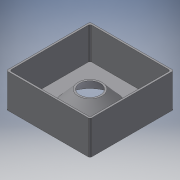
# Autodesk Inventor part: contenção
Saved by Autodesk Inventor 2019.4 (Build 234330000, 330)
## iProperties
Created: 2019-10-16
Part Number: contenção
Material: Genérico
Document SubType Name: Modeling
Designer: natha
Density: 1 g/cm^3
Appearance: Padrão
Author: natha
Autodesk Inventor part; units mm, degrees
ref_plane "YZ Plane" through (0, 0, 0) normal (1, 0, 0) x (0, 1, 0)
ref_plane "XY Plane" through (0, 0, 0) normal (0, 0, 1) x (1, 0, 0)
sketch "Esboço1" plane through (0, 0, 0) normal (0, 1, 0) x (-1, 0, 0)
  line L0 (-49, 49) -> (49, 49)
  line L1 (49, 49) -> (49, -49)
  line L2 (49, -49) -> (-49, -49)
  line L3 (-49, -49) -> (-49, 49)
  line L4 (-49, 49) -> (49, -49) construction
  line L5 (49, 49) -> (-49, -49) construction
  point P0 (0, 0)
  dimension "d0" = 98
  dimension "d1" = 98
  constraints: 12 end point, 2 midpoint, 2 parallel, 1 horizontal, 1 perpendicular
  measures "d0" distance of L0.end L1.end
  measures "d1" distance of L1.end L2.end
extrude "Extrusão1" add sketch "Esboço1" along normal blind 39.4
shell "Casca1" thickness 2 removed faces 1 at (16.3333, 39.4, 16.3333)
sketch "Esboço3" plane through (0, 0, 0) normal (0, 0, 1) x (1, 0, 0)
  line L0 (0, 0) -> (32, 0)
  line L1 (49, 0) -> (-49, 0) projected
  line L2 (32, 0) -> (0, 36.5533)
  line L3 (0, 0) -> (0, 36.5533)
  point P0 (-43.1, 0)
  dimension "d6" = 32
  dimension "d7" = 48.8
  constraints: 6 end point, 1 point on line, 1 vertical
  measures "d6" distance of L0.start L0.end
  measures "d7" angle of L0 L2
revolve "Revolução1" add sketch "Esboço3" angle 360 about axis through (0, 0, 0) along (0, 1, 0)
sketch "Esboço4" plane through (0, 0, 0) normal (0, 0, 1) x (1, 0, 0)
  line L0 (0, 0) -> (30, 0)
  line L1 (-49, 0) -> (49, 0) projected
  line L2 (0, 36.5533) -> (-30.2491, 2) projected
  line L3 (30, 0) -> (0, 34.2687)
  line L4 (0, 0) -> (0, 34.2687)
  point P0 (43.1, 0)
  dimension "d9" = 30
  dimension "d10" = 48.8
  constraints: 6 end point, 1 point on line, 1 vertical
  measures "d9" distance of L0.start L0.end
  measures "d10" angle of L0 L3
revolve "Revolução2" cut sketch "Esboço4" angle 360 about axis through (0, 0, 0) along (0, 1, 0)
ref_plane "Plano de trabalho1" through (0, 39.4, 0) normal (0, 1, 0) x (-1, 0, 0)
sketch "Esboço5" plane through (0, 39.4, 0) normal (0, 1, 0) x (-1, 0, 0)
  line L0 (31.6566, 29.5617) -> (-31.6566, 29.5617)
  line L1 (-31.6566, 29.5617) -> (-31.6566, -29.5617)
  line L2 (-31.6566, -29.5617) -> (31.6566, -29.5617)
  line L3 (31.6566, -29.5617) -> (31.6566, 29.5617)
  line L4 (31.6566, 29.5617) -> (-31.6566, -29.5617) construction
  line L5 (-31.6566, 29.5617) -> (31.6566, -29.5617) construction
  point P0 (0, 0)
  constraints: 12 end point, 2 midpoint, 2 parallel, 1 horizontal, 1 perpendicular
extrude "Extrusão2" cut sketch "Esboço5" against normal blind 18.8
sketch "Esboço6" plane through (0, 0, 0) normal (0, 1, 0) x (-1, 0, 0)
  point P0 (0, 0)
fillet "Arredondamento2" radius 2 8 edges at (47, 20.7, 47) (49, 19.7, 49) (-47, 20.7, 47) (-49, 19.7, 49) (-49, 19.7, -49) (-47, 20.7, -47) (49, 19.7, -49) (47, 20.7, -47)
